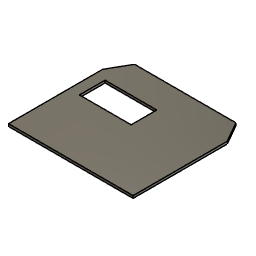
Bauwagen Seite Deichsel MK1 v3 (Autodesk Fusion 360 design; units mm, degrees)
Autodesk Fusion 360 part; units mm, degrees
sketch "Skizze1" plane through (0, 0, 0) normal (0, 1, 0) x (1, 0, 0)
  line L0 (0, 0) -> (258, 0)
  line L1 (258, 0) -> (258, 237)
  line L2 (0, 0) -> (0, 185)
  line L3 (0, 185) -> (258, 185)
  line L4 (258, 237) -> (0, 237)
  line L5 (0, 237) -> (0, 185)
  line L6 (0, 185) -> (24.5, 185)
  line L7 (258, 185) -> (233.5, 185)
  line L8 (24.5, 237) -> (233.5, 237)
  line L9 (0, 185) -> (24.5, 237)
  line L10 (258, 185) -> (233.5, 237)
  dimension "d1" = 258
  dimension "d2" = 237
  dimension "d3" = 185
  dimension "d4" = 24.5
  dimension "d5" = 24.5
  dimension "d6" = 209
  constraint coincident L0.start L2.start
  constraint horizontal L0
  constraint perpendicular L0 L1
  constraint perpendicular L0 L2
  constraint coincident L1 L3.end
  constraint perpendicular L1 L3
  constraint perpendicular L1 L4
  constraint perpendicular L4 L5
  constraint perpendicular L5 L6
  constraint perpendicular L1 L7
  constraint coincident L4 L8.start
  constraint parallel L4 L8
  measures "d1" distance of L0.start L0.end
  measures "d2" distance of L0.end L1.end
  measures "d3" distance of L0.start L2.end
  measures "d4" distance of L2.end L6.end
  measures "d5" distance of L3.end L7.end
  measures "d6" distance of L8.start L8.end
  measures "d10" distance of L0.start
  measures "d11" distance of L0.start
  measures "d12" distance of L0.start
  measures "d25" distance of L0.start
extrude "Extrusion1" add sketch "Skizze1" along normal blind 5 contours L0 L1 L2 L3 L6 L7 | L3 L4 L6 L7 L8 L9 L10
sketch "Skizze2" plane through (0, 5, 0) normal (0, 1, 0) x (-1, 0, 0)
  line L0 (0, 0) -> (-258, 0)
  line L1 (-258, 0) -> (-258, -185)
  line L2 (-258, -185) -> (-233.5, -237)
  line L3 (-233.5, -237) -> (-24.5, -237)
  line L4 (-24.5, -237) -> (0, -185)
  line L5 (0, -185) -> (0, 0)
  line L6 (0, -185) -> (-258, -185)
  line L7 (0, 0) -> (0, -125)
  line L8 (0, -125) -> (-22, -125)
  line L9 (-22, -125) -> (-129, -125)
  line L10 (-129, -125) -> (-129, -178)
  line L11 (-129, -178) -> (-22, -178)
  line L12 (-22, -178) -> (-22, -125)
  dimension "d9" = 125
  dimension "d10" = 22
  dimension "d11" = 107
  dimension "d12" = 53
  constraint coincident L4.end L5.start
  constraint coincident L1.end L2.start
  constraint coincident L0.start L5.end
  constraint perpendicular L0 L7
  constraint perpendicular L7 L8
  constraint horizontal L9
  constraint vertical L10
  constraint horizontal L11
  constraint vertical L12
  measures "d9" distance of L0.start L7.end
  measures "d10" distance of L7.end L8.end
  measures "d11" distance of L8.end L9.end
  measures "d12" distance of L8.end L11.end
extrude "Extrusion2" cut sketch "Skizze2" against normal blind 50 contours L9 L10 L11 L12
sketch "Skizze3" plane through (0, 5, 0) normal (0, 1, 0) x (-1, 0, 0)
  line L0 (-129, -125) -> (-22, -125)
  line L1 (-22, -125) -> (-22, -178)
  line L2 (-22, -178) -> (-129, -178)
  line L3 (-129, -178) -> (-129, -125)
  line L4 (0, 0) -> (-258, 0)
  line L5 (-258, 0) -> (-258, -185)
  line L6 (-258, -185) -> (-233.5, -237)
  line L7 (-233.5, -237) -> (-24.5, -237)
  line L8 (-24.5, -237) -> (0, -185)
  line L9 (0, -185) -> (0, 0)
  line L10 (0, -185) -> (-30.8644, -237)
  line L11 (-258, -185) -> (-230, -237)
  constraint coincident L8.end L9.start
  constraint coincident L7 L10.end
  constraint coincident L5.end L6.start
  constraint coincident L7 L11.end
extrude "Extrusion3" cut sketch "Skizze3" against normal blind 30 contours L7 L8 L10 | L6 L7 L11
sketch "Skizze4" plane through (0, 5, 0) normal (0, 1, 0) x (-1, 0, 0)
  line L0 (-30.8644, -237) -> (0, -185)
  line L1 (0, -185) -> (0, 0)
  line L2 (0, 0) -> (-258, 0)
  line L3 (-258, 0) -> (-258, -185)
  line L4 (-258, -185) -> (-230, -237)
  line L5 (-230, -237) -> (-30.8644, -237)
  line L6 (-129, -125) -> (-22, -125)
  line L7 (-22, -125) -> (-22, -178)
  line L8 (-22, -178) -> (-129, -178)
  line L9 (-129, -178) -> (-129, -125)
  line L10 (-30.8644, -237) -> (0, -237)
  line L11 (0, -237) -> (0, -185)
  line L12 (-258, -185) -> (-258, -237)
  line L13 (-258, -237) -> (-230, -237)
  constraint coincident L0.start L5.end
  constraint parallel L5 L10
  constraint coincident L0.end L1.start
  constraint perpendicular L10 L11
  constraint coincident L3.end L4.start
  constraint parallel L3 L12
  constraint coincident L4.end L5.start
  constraint perpendicular L3 L13
extrude "Extrusion4" add sketch "Skizze4" against normal blind 5 contours L0 L10 L11 | L4 L12 L13
sketch "Skizze5" plane through (0, 5, 0) normal (0, 1, 0) x (-1, 0, 0)
  line L0 (0, -237) -> (0, 0)
  line L1 (0, 0) -> (-258, 0)
  line L2 (-258, 0) -> (-258, -237)
  line L3 (-258, -237) -> (-230, -237)
  line L4 (-230, -237) -> (0, -237)
  line L5 (-129, -125) -> (-22, -125)
  line L6 (-22, -125) -> (-22, -178)
  line L7 (-22, -178) -> (-129, -178)
  line L8 (-129, -178) -> (-129, -125)
  line L9 (0, -237) -> (-24, -237)
  line L10 (-258, -237) -> (-234, -237)
  line L11 (0, -237) -> (0, -187)
  line L12 (-258, -237) -> (-258, -187)
  line L13 (0, -187) -> (-24, -237)
  line L14 (-258, -187) -> (-234, -237)
  dimension "d19" = 24
  dimension "d20" = 24
  dimension "d21" = 50
  dimension "d22" = 50
  constraint coincident L0.start L4.end
  constraint perpendicular L0 L9
  constraint coincident L2.end L3.start
  constraint perpendicular L2 L10
  constraint perpendicular L4 L11
  constraint perpendicular L3 L12
  measures "d19" distance of L0.start L9.end
  measures "d20" distance of L2.end L10.end
  measures "d21" distance of L0.start L11.end
  measures "d22" distance of L2.end L12.end
extrude "Extrusion5" cut sketch "Skizze5" against normal blind 45 contours L0 L4 L9 L11 L13 | L2 L3 L10 L12 L14
sketch "Skizze6" plane through (0, 5, 0) normal (0, 1, 0) x (-1, 0, 0)
  line L0 (-24, -237) -> (0, -187)
  line L1 (0, -187) -> (0, 0)
  line L2 (0, 0) -> (-258, 0)
  line L3 (-258, 0) -> (-258, -187)
  line L4 (-258, -187) -> (-234, -237)
  line L5 (-234, -237) -> (-230, -237)
  line L6 (-230, -237) -> (-24, -237)
  line L7 (-129, -125) -> (-22, -125)
  line L8 (-22, -125) -> (-22, -178)
  line L9 (-22, -178) -> (-129, -178)
  line L10 (-129, -178) -> (-129, -125)
  line L11 (0, 0) -> (0, -195)
  line L12 (-258, 0) -> (-258, -195)
  line L13 (0, -195) -> (-24, -237)
  line L14 (-258, -195) -> (-234, -237)
  dimension "d25" = 195
  dimension "d26" = 195
  constraint coincident L1.end L2.start
  constraint perpendicular L2 L11
  constraint coincident L2.end L3.start
  constraint perpendicular L2 L12
  constraint coincident L0.start L6.end
  constraint coincident L4.end L5.start
  measures "d25" distance of L1.end L11.end
  measures "d26" distance of L2.end L12.end
extrude "Extrusion6" add sketch "Skizze6" against normal blind 5 contours L0 L11 L13 | L4 L12 L14
